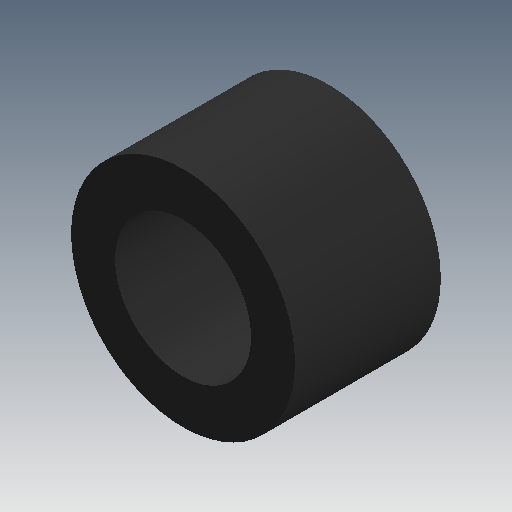
# Autodesk Inventor part: Bushing
Saved by Autodesk Inventor 2020 (Build 240168000, 168)
## iProperties
Created: 2019-05-22
Part Number: Bushing
Material: Rubber
Document SubType Name: Modeling
Designer: chitl
Density: 0.93 g/cm^3
Appearance: Rubber - Black
Mass: 0.0768624 g
Surface Area: 1.72735 cm^2
Volume: 0.0826477 cm^3
Author: chitl
Autodesk Inventor part; units mm, degrees
ref_plane "YZ Plane" through (0, 0, 0) normal (1, 0, 0) x (0, 1, 0)
ref_plane "XZ Plane" through (0, 0, 0) normal (0, 1, 0) x (-1, 0, 0)
ref_plane "XY Plane" through (0, 0, 0) normal (0, 0, 1) x (1, 0, 0)
sketch "Sketch1" plane through (0, 0, 0) normal (0, 0, 1) x (1, 0, 0)
  circle A0 centre (0, 0) radius 3.175
  dimension "d0" = 6.35
  constraints: 1 centre point, 1 coincident
  measures "d0" diameter of A0
extrude "Extrusion1" add sketch "Sketch1" along normal blind 4.1402
sketch "Sketch2" plane through (0, 0, 4.1402) normal (0, 0, 1) x (1, 0, 0)
  point P0 (0, 0)
  point P1 (0, 0)
  constraints: 1 coincident
hole "Hole1" at (0, 0, 4.1402) direction (0, 0, -1) diameter 3.8608 depth 95.25 tip angle 118
body "Solid1"
